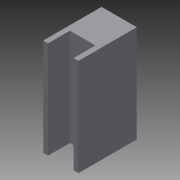
# Autodesk Inventor part: bloc
Saved by Autodesk Inventor 2014 (Build 180170000, 170)
## iProperties
Created: 2014-01-16
Part Number: bloc
Material: Générique
Document SubType Name: Modeling
Designer: helly
Density: 1 g/cm^3
Appearance: Par défaut
Author: helly
Autodesk Inventor part; units mm, degrees
ref_plane "YZ Plane" through (0, 0, 0) normal (1, 0, 0) x (0, 1, 0)
ref_plane "XZ Plane" through (0, 0, 0) normal (0, 1, 0) x (-1, 0, 0)
ref_plane "XY Plane" through (0, 0, 0) normal (0, 0, 1) x (1, 0, 0)
sketch "Esquisse1" plane through (0, 0, 0) normal (0, 0, 1) x (1, 0, 0)
  line L0 (0, 0) -> (0, 15)
  line L1 (0, 15) -> (10.5, 15)
  line L2 (10.5, 15) -> (10.5, 0)
  line L3 (10.5, 0) -> (0, 0)
  line L4 (10.5, 15) -> (12.5, 15)
  line L5 (0, 15) -> (-2, 15)
  line L6 (-2, 15) -> (-2, -9)
  line L7 (-2, -9) -> (0, -9)
  line L8 (0, -9) -> (0, 0)
  line L9 (12.5, 15) -> (12.5, -9)
  line L10 (12.5, -9) -> (10.5, -9)
  line L11 (10.5, -9) -> (10.5, 0)
  dimension "d0" = 15
  dimension "d1" = 10.5
  dimension "d7" = 2
  dimension "d8" = 2
  dimension "d10" = 9
  constraints: 24 end point, 7 parallel, 4 perpendicular, 1 collinear, 1 vertical
  measures "d0" distance of L0.start L0.end
  measures "d1" distance of L0.end L1.end
  measures "d7" distance of L0.end L5.end
  measures "d8" distance of L1.end L4.end
  measures "d10" distance of L7.end L0.start
extrude "Extrusion2" add sketch "Esquisse1" along normal blind 40
